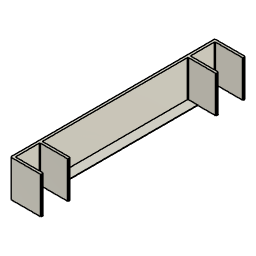
MERV-Filter-Flat-Joiner v13 (Autodesk Fusion 360 design; units mm, degrees)
Autodesk Fusion 360 part; units mm, degrees
sketch "Sketch1" plane through (0, 0, 0) normal (0, 1, 0) x (1, 0, 0)
  line L0 (0, 0) -> (30, 0)
  line L1 (30, 0) -> (30, -25)
  line L2 (30, -25) -> (0, -25)
  line L3 (0, -25) -> (0, 0)
  line L4 (30, -2) -> (0, -2)
  line L5 (29, 0) -> (29, -25)
  dimension "d1" = 30
  dimension "d2" = 25
  dimension "d3" = 2
  dimension "d4" = 1
  constraint horizontal L0
  constraint vertical L1
  constraint horizontal L2
  constraint vertical L3
  constraint coincident L0.start L3.end
  constraint coincident L1 L4.start
  constraint coincident L3 L4.end
  constraint perpendicular L3 L4
  constraint coincident L0 L5.start
  constraint coincident L2 L5.end
  constraint perpendicular L2 L5
  measures "d1" distance of L0.start L0.end
  measures "d2" distance of L0.start L2.end
  measures "d3" distance of L0 L4
  measures "d4" distance of L1 L5
extrude "Extrude1" add sketch "Sketch1" along normal blind 2
extrude "Extrude2" add sketch "Sketch1" along normal blind 167 contours L0 L3 L4 L5 | L0 L1 L4 L5
extrude "Extrude3" add sketch "Sketch1" along normal blind 2 from surface at 22
extrude "Extrude4" add sketch "Sketch1" against normal blind 2 from surface at 167
extrude "Extrude5" add sketch "Sketch1" against normal blind 2 from surface at 145
sketch "Sketch2" plane through (30, 0, 0) normal (1, 0, 0) x (0, 1, 0)
  line L0 (0, 25) -> (0, 0)
  line L1 (0, 0) -> (167, 0)
  line L2 (167, 0) -> (167, 25)
  line L3 (167, 25) -> (165, 25)
  line L4 (165, 25) -> (165, 2)
  line L5 (165, 2) -> (145, 2)
  line L6 (145, 2) -> (145, 25)
  line L7 (145, 25) -> (143, 25)
  line L8 (143, 25) -> (143, 2)
  line L9 (24, 2) -> (24, 25)
  line L10 (24, 25) -> (22, 25)
  line L11 (22, 25) -> (22, 2)
  line L12 (2, 2) -> (2, 25)
  line L13 (2, 25) -> (0, 25)
  line L14 (24, 25) -> (143, 25)
  line L15 (143, 25) -> (143, 1.5)
  line L16 (143, 1.5) -> (24, 1.5)
  line L17 (24, 1.5) -> (24, 25)
  line L18 (24, 10) -> (143, 10)
  line L19 (143, 2) -> (24, 2)
  line L20 (22, 2) -> (2, 2)
  constraint horizontal L14
  constraint vertical L15
  constraint horizontal L16
  constraint vertical L17
  constraint coincident L9.end L10.start
  constraint coincident L17 L18.start
  constraint coincident L15 L18.end
  constraint perpendicular L15 L18
extrude "Extrude6" add sketch "Sketch2" against normal blind 0.3 contours L8 L9 L15 L17 L18 L19
fillet "Fillet1" radius 0.5 18 edges at (15, 167, 0) (15, 165, 2) (15, 0, 0) (15, 2, 2) (15, 22, 2) (15, 145, 2) (15, 167, 25) (15, 165, 25) (15, 145, 25) (15, 143, 25) (15, 24, 25) (15, 22, 25) (15, 2, 25) (15, 0, 25) (14.85, 24, 2) (14.85, 143, 2) (29.85, 143, 10) (29.85, 24, 10)
move_body "Move1" bodies 1 to x (0, 0, -1) y (0, 1, 0) z (1, 0, 0) at (30, 0, 30)
equation "d1 = length"
equation "d2 = height"
equation "length = 30 mm"
equation "height = 25 mm"
